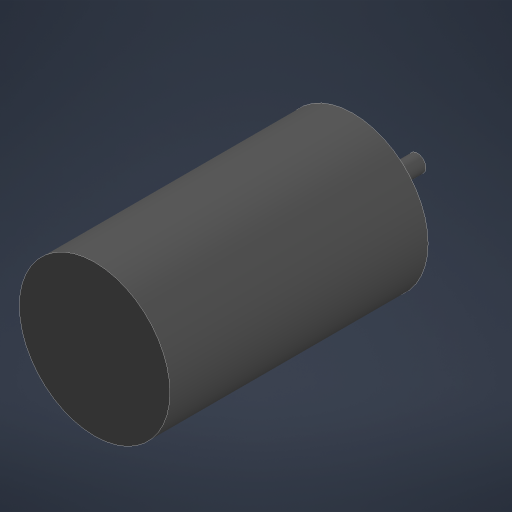
# Autodesk Inventor part: motor
Saved by Autodesk Inventor 2023 (Build 270158030, 158C)
## iProperties
Created: 2022-03-30
Part Number: motor
Material: Generic
Document SubType Name: Modeling
Designer: kardo
Density: 1 g/cm^3
Appearance: Dark Plastic
Mass: 30.8826 g
Surface Area: 57.4943 cm^2
Volume: 30.8826 cm^3
Author: kardo
Autodesk Inventor part; units mm, degrees
ref_plane "YZ Plane" through (0, 0, 0) normal (1, 0, 0) x (0, 1, 0)
ref_plane "XZ Plane" through (0, 0, 0) normal (0, 1, 0) x (-1, 0, 0)
ref_plane "XY Plane" through (0, 0, 0) normal (0, 0, 1) x (1, 0, 0)
derived "parameters_powertrain.ipt"
sketch "sk_section" plane through (0, 0, 0) normal (0, 0, 1) x (1, 0, 0)
  circle A0 centre (0, 0) radius 14
  dimension "d1" = 28
  constraints: 1 centre point, 1 coincident
  measures "d1" diameter of A0
sketch "sk_shaft" plane through (0, 0, 0) normal (0, 0, 1) x (1, 0, 0)
  circle A0 centre (0, 0) radius 1.5875
  dimension "d2" = 3.175
  constraints: 1 centre point, 1 coincident
  measures "d2" diameter of A0
extrude "body" add sketch "sk_section" along normal blind 48
extrude "shaft" add sketch "sk_shaft" against normal blind 12
equation "\"d1\" = motor_diameter"
equation "\"motor_diameter\" = 28"
body "Solid1"
